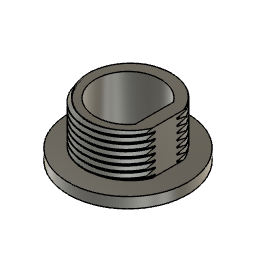
DoubleSHVFeedthroughFilterUsingAdapters (Autodesk Fusion 360 archive; units mm, degrees)
design "SHVBulkheadAdapter"
Autodesk Fusion 360 part; units mm, degrees
sketch "Sketch1" plane through (0, 0, 0) normal (0, 0, 1) x (1, 0, 0)
  circle A0 centre (0, 0) radius 8.7122
  circle A1 centre (0, 0) radius 4.7625
  line L0 (3.8481, 2.806) -> (3.8481, -2.806)
  dimension "d1" = 17.4244
  dimension "d2" = 9.525
  dimension "d3" = 3.8481
  constraint coincident A0.centre A1.centre
  constraint concentric A0 A1
  constraint coincident A1 L0.start
  constraint coincident A1 L0.end
  constraint vertical L0
  measures "d1" diameter of A0
  measures "d2" diameter of A1
  measures "d3" distance of A0.centre L0
extrude "Extrude1" add sketch "Sketch1" along normal blind 7.8994 contours A0 | A1 L0 picked at (3.9555, -0.7667)
sketch "Sketch2" plane through (0, 0, 7.8994) normal (0, 0, 1) x (-1, 0, 0)
  arc A0 (-3.8481, -2.806) -> (-3.8481, 2.806) centre (0, 0) ccw
  line L0 (-3.8481, -2.806) -> (-3.8481, 2.806)
  circle A1 centre (0, 0) radius 8.7122
  circle A2 centre (0, 0) radius 6.35
  line L1 (-5.588, -3.0161) -> (-5.588, 3.0161)
  dimension "d6" = 12.7
  dimension "d7" = 5.588
  constraint coincident A0.centre A1.centre
  constraint coincident A2 L1.start
  constraint coincident A2 L1.end
  constraint parallel L0 L1
  measures "d6" diameter of A2
  measures "d7" distance of A0.centre L1
extrude "Extrude2" cut sketch "Sketch2" against normal blind 6.35 contours A1 | A2 L1 picked at (-5.7111, 0.7328)
thread "Thread1" "ANSI Unified Screw Threads 0.5 1/2-28 UNEF 3A" major diameter 12.6187 minor diameter 11.618 pitch 0.9071 angle 60 modelled right hand crest width 0.1397 on face at (5.4335, 3.2862, 5.7827) crest through (-6.3094, 0, 8.1262)
equation "d1 = 0.75 in - 0.064 in"
equation "d3 = 0.339 in - 0.375 in / 2"
equation "d7 = 0.47 in - 0.25 in"

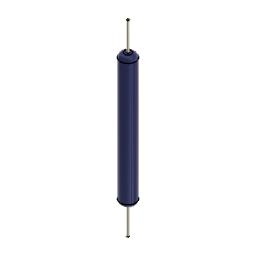
design "MOX1125-22"
Autodesk Fusion 360 part; units mm, degrees
sketch "Sketch1" plane through (0, 0, 0) normal (0, 0, 1) x (1, 0, 0)
  circle A0 centre (0, 0) radius 1.78
  dimension "d1" = 3.56
  constraint coincident A0.centre origin
  measures "d1" diameter of A0
extrude "Extrude1" add sketch "Sketch1" along normal mid plane 30.73 makes body 1
sketch "Sketch2" plane through (0, 0, 15.365) normal (0, 0, 1) x (-1, 0, 0)
  circle A0 centre (0, 0) radius 1.78
  circle A1 centre (0, 0) radius 0.254
  dimension "d4" = 0.508
  constraint concentric A0 A1
  measures "d4" diameter of A1
extrude "Extrude2" add sketch "Sketch2" along normal blind 6.63 separate body contours A1 makes body 2
mirror "Mirror1" about plane through (0, 0, 0) normal (0, 0, 1) of "Extrude2" makes body 3
fillet "Fillet1" radius 1 2 edges at (-1.6595, -0.6437, 15.365) (-1.6595, 0.6437, -15.365) on bodies 1
equation "d2 = 30.73 mm / 2"

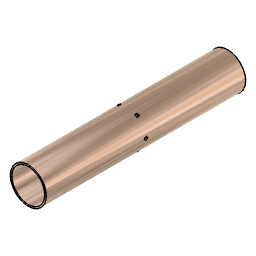
design "OuterTubeLong"
Autodesk Fusion 360 part; units mm, degrees
sketch "Sketch1" plane through (0, 0, 0) normal (0, 1, 0) x (1, 0, 0)
  circle A0 centre (0, 0) radius 9.525
  circle A1 centre (0, 0) radius 8.7122
  dimension "d1" = 19.05
  dimension "d2" = 0.8128
  constraint coincident A0.centre A1.centre
  constraint concentric A0 A1
  measures "d1" diameter of A0
  measures "d2" distance of A0 A1
extrude "Extrude1" add sketch "Sketch1" along normal mid plane 105.6
sketch "Sketch2" plane through (0, 0, 0) normal (1, 0, 0) x (0, 1, 0)
hole "Hole1" at (0, 0, 0) direction (-1, 0, 0) diameter 1.5875 end through all
pattern_circular "C-Pattern2" count 6 over 360 about axis through (0, 1.75, 0) along (0, 1, 0) of "Hole1"
sketch "Sketch3" plane through (0, 0, 0) normal (1, 0, 0) x (0, 1, 0)
  line L0 (52.8, -9.525) -> (52.8, 9.525)
  point P0 (50.06, 0)
  dimension "d12" = 2.74
  constraint horizontal origin P0
  measures "d12" distance of P0 L0
hole "Hole2" at (0, 50.06, 0) direction (-1, 0, 0) diameter 2.3813 end through all
equation "d6 = 1 in / 16"
equation "d12 = 0.061 in + 3 in / 64"
equation "d14 = 3 in / 32"

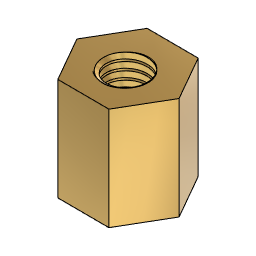
design "CapacitorArrayCenter"
Autodesk Fusion 360 part; units mm, degrees
sketch "Sketch1" plane through (0, 0, 0) normal (0, 0, 1) x (1, 0, 0)
  line L0 (1.5999, 2.7429) -> (-1.5755, 2.757)
  line L1 (-1.5755, 2.757) -> (-3.1754, 0.0141)
  line L2 (-3.1754, 0.0141) -> (-1.5999, -2.7429)
  line L3 (-1.5999, -2.7429) -> (1.5755, -2.757)
  line L4 (1.5755, -2.757) -> (3.1754, -0.0141)
  line L5 (3.1754, -0.0141) -> (1.5999, 2.7429)
  dimension "d1" = 5.5
  measures "d1" distance of L0 L3
extrude "Extrude1" add sketch "Sketch1" along normal mid plane 6.35
sketch "Sketch2" plane through (0, 0, 3.175) normal (0, 0, 1) x (-1, 0, 0)
  line L0 (-3.1754, 0.0141) -> (-1.5999, -2.7429)
  line L1 (-1.5999, -2.7429) -> (1.5755, -2.757)
  line L2 (1.5755, -2.757) -> (3.1754, -0.0141)
  line L3 (3.1754, -0.0141) -> (1.5999, 2.7429)
  line L4 (1.5999, 2.7429) -> (-1.5755, 2.757)
  line L5 (-1.5755, 2.757) -> (-3.1754, 0.0141)
hole "Hole1" at (0, 0, 3.175) direction (0, 0, -1) diameter 2.529 end through all
thread "Thread1" "ISO Metric profile 3.0 M3x0.5 6H" major diameter 3.086 minor diameter 2.529 pitch 0.5 angle 60 modelled right hand crest width 0.1368 on face at (0.1259, -1.2582, 1.0583) crest through (1.2645, 0, 3.05)
